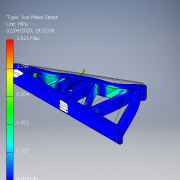
# Autodesk Inventor part: SupportArm
Saved by Autodesk Inventor 2018.3 (Build 223284000, 284)
## iProperties
Created: 2020-04-02
Part Number: SupportArm
Material: Generic
Document SubType Name: Modeling
Designer: Ivan
Density: 1 g/cm^3
Appearance: Default
Author: Ivan
Autodesk Inventor part; units mm, degrees
ref_plane "YZ Plane" through (0, 0, 0) normal (1, 0, 0) x (0, 1, 0)
ref_plane "XZ Plane" through (0, 0, 0) normal (0, 1, 0) x (-1, 0, 0)
sketch "Sketch1" plane through (0, 0, 0) normal (0, 0, 1) x (1, 0, 0)
  line L0 (0, 0) -> (130, 0)
  line L1 (130, 0) -> (130, 6)
  line L2 (130, 6) -> (0, 6)
  line L3 (0, 6) -> (0, 0)
  line L4 (0, 6) -> (99.592921, 63.5)
  line L5 (99.592921, 63.5) -> (96.592921, 68.696152)
  line L6 (96.592921, 68.696152) -> (-3, 11.196152)
  line L7 (-3, 11.196152) -> (0, 6)
  circle A0 centre (0, 6) radius 6
  dimension "d0" = 130
  dimension "d1" = 6
  dimension "d2" = 6
  dimension "d47" = 30
  dimension "d57" = 115
  constraints: 16 end point, 4 parallel, 3 coincident, 2 perpendicular, 1 centre point, 1 horizontal, 1 tangent
  measures "d0" distance of L2.end L1.end
  measures "d1" distance of L1.end L0.end
  measures "d2" distance of L5.end L4.end
  measures "d47" angle of L2 L4
  measures "d57" distance of L5.end L6.end
extrude "Extrusion1" add sketch "Sketch1" along normal blind 15
fillet "Fillet1" radius 2 3 edges at (130, 6, 7.5) (99.5929, 63.5, 7.5) (96.5929, 68.6962, 7.5)
fillet "Fillet2" radius 2 14 edges at (98.7927, 63.7144, 15) (98.0929, 66.0981, 15) (96.3785, 67.896, 15) (45.9304, 39.4462, 15) (-5.7956, 4.4471, 15) (65, 0, 15) (51.5285, 35.75, 15) (98.7927, 63.7144, 0) (98.0929, 66.0981, 0) (96.3785, 67.896, 0) (45.9304, 39.4462, 0) (-5.7956, 4.4471, 0) (65, 0, 0) (51.5285, 35.75, 0)
fillet "Fillet3" radius 2 5 edges at (4.614, 9.8355, 15) (5.7956, 7.5529, 15) (5.7956, 7.5529, 0) (4.614, 9.8355, 0) (6, 6, 7.5)
ref_plane "Work Plane1" through (0, 0, 7.5) normal (0, 0, 1) x (1, 0, 0)
sketch "Sketch2" plane through (0, 0, 7.5) normal (0, 0, 1) x (1, 0, 0)
  line L0 (5.196152, 9) -> (97.860871, 62.5) construction
  line L1 (128, 6) -> (7.191162, 6) construction
  line L2 (22.191162, 6) -> (16.643372, 15.609055)
  line L3 (22.191162, 6) -> (35.70691, 6) construction
  line L4 (16.643372, 15.609055) -> (33.286743, 6)
  line L5 (16.643372, 15.609055) -> (35.861482, 15.609055) construction
  line L6 (33.286743, 6) -> (50.034147, 6) construction
  line L7 (37.720378, 6) -> (61.042821, 6) construction
  line L8 (36.286743, 6) -> (18.143372, 16.47508)
  line L9 (14.561151, 14.406884) -> (19.414868, 6)
  line L10 (36.286743, 6) -> (33.286743, 6)
  line L11 (16.643372, 15.609055) -> (18.143372, 16.47508)
  line L12 (16.643372, 15.609055) -> (14.561151, 14.406884)
  line L13 (19.414868, 6) -> (22.191162, 6)
  line L14 (36.286743, 6) -> (36.286743, 26.950161)
  line L15 (36.286743, 6) -> (57.236904, 6) construction
  line L16 (36.286743, 26.950161) -> (79.251589, 26.950161) construction
  line L17 (36.286743, 6) -> (36.220378, 6)
  line L18 (66.440756, 6) -> (69.440756, 6)
  line L19 (69.440756, 6) -> (111.994218, 6) construction
  line L20 (69.440756, 6) -> (72.440756, 6)
  line L21 (39.286743, 6) -> (39.286743, 28.682212)
  line L22 (39.286743, 28.682212) -> (52.382324, 6)
  line L23 (39.286743, 28.682212) -> (65.477905, 28.682212) construction
  line L24 (41.884819, 30.182212) -> (55.846426, 6)
  line L25 (55.846426, 6) -> (55.846426, 38.242949)
  line L26 (97.860871, 62.5) -> (5.196152, 9)
  line L27 (55.846426, 6) -> (88.089375, 6) construction
  line L28 (59.846426, 6) -> (59.846426, 40.55235)
  line L29 (52.382324, 6) -> (55.846426, 6)
  line L30 (128, 6) -> (7.191162, 6)
  line L31 (55.846426, 6) -> (59.846426, 6)
  line L32 (39.286743, 28.682212) -> (41.884819, 30.182212)
  line L33 (39.286743, 28.682212) -> (36.286743, 26.950161)
  line L34 (36.286743, 6) -> (39.286743, 6)
  line L35 (33.286743, 6) -> (36.286743, 6)
  line L36 (59.846426, 40.55235) -> (98.351719, 40.55235) construction
  line L37 (90.414037, 58.200568) -> (120.552049, 6)
  line L38 (90.414037, 58.200568) -> (150.690061, 58.200568) construction
  line L39 (127.480252, 6) -> (95.610189, 61.200568)
  line L40 (127.480252, 6) -> (120.552049, 6)
  line L41 (90.414037, 58.200568) -> (95.610189, 61.200568)
  line L42 (59.846426, 40.55235) -> (55.846426, 38.242949)
  line L43 (59.846426, 40.55235) -> (63.310528, 42.55235)
  line L44 (63.310528, 42.55235) -> (84.414037, 6)
  line L45 (59.846426, 40.55235) -> (79.795235, 6)
  line L46 (84.414037, 6) -> (79.795235, 6)
  line L47 (84.414037, 6) -> (90.414037, 6)
  line L48 (90.414037, 6) -> (90.414037, 58.200568)
  line L49 (90.414037, 58.200568) -> (84.414037, 54.736467)
  line L50 (84.414037, 54.736467) -> (84.414037, 6)
  line L51 (33.286743, 6) -> (36.220378, 6)
  line L52 (16.643372, 15.609055) -> (18.143372, 16.47508)
  point P0 (0, 0)
  dimension "d8" = 120
  dimension "d9" = 15
  dimension "d10" = 30
  dimension "d15" = 1.5
  dimension "d18" = 90
  dimension "d28" = 3
  dimension "d29" = 60
  dimension "d30" = 3
  dimension "d31" = 90
  dimension "d32" = 4
  dimension "d51" = 60
  dimension "d52" = 6
  dimension "d54" = 6
  dimension "d55" = 4
  dimension "d56" = 60
  constraints: 98 end point, 17 point on line, 15 horizontal, 14 collinear, 5 equal length, 3 parallel, 1 perpendicular, 1 vertical, 14 other
  measures "d8" angle of L3 L2
  measures "d9" distance of L2.start L1.end
  measures "d10" angle of L4 L5
  measures "d15" distance between parallel lines of L4 L8
  measures "d18" angle of L15 L14
  measures "d28" distance between parallel lines of L14 L21
  measures "d29" angle of L22 L23
  measures "d30" distance between parallel lines of L22 L24
  measures "d31" angle of L27 L25
  measures "d32" distance between parallel lines of L25 L28
  measures "d51" angle of L37 L38
  measures "d52" distance between parallel lines of L37 L39
  measures "d54" distance between parallel lines of L50 L48
  measures "d55" distance between parallel lines of L45 L44
  measures "d56" angle of L36 L44
extrude "Extrusion5" add sketch "Sketch2" along normal mid plane 10 contours L13 L9 L12 L2 | L11 L8 L10 L4 | L14 L26 L21 L30 | L26 L24 L29 L22 | L25 L26 L28 L30 | L26 L44 L30 L45 | L26 L48 L30 L50 | L26 L39 L30 L37
body "Solid1"
